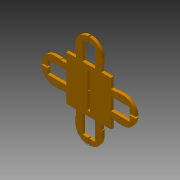
# Autodesk Inventor part: Lock2
Saved by Autodesk Inventor 2014 SP2 (Build 180246200, 246)
## iProperties
Created: 2014-11-24
Part Number: Lock2
Material: Generic
Document SubType Name: Modeling
Designer: JLM
Density: 1 g/cm^3
Appearance: Default
Author: JLM
Autodesk Inventor part; units mm, degrees
ref_plane "YZ Plane" through (0, 0, 0) normal (1, 0, 0) x (0, 1, 0)
ref_plane "XZ Plane" through (0, 0, 0) normal (0, 1, 0) x (-1, 0, 0)
ref_plane "XY Plane" through (0, 0, 0) normal (0, 0, 1) x (1, 0, 0)
sketch "Sketch1" plane through (0, 0, 0) normal (0, 0, 1) x (1, 0, 0)
  line L0 (47.1932, 0) -> (47.1932, 13.335)
  line L1 (47.1932, 13.335) -> (28.1432, 13.335)
  line L2 (28.1432, 13.335) -> (28.1432, 12.7)
  line L3 (28.1432, 12.7) -> (22.4282, 12.7)
  line L4 (12.2521, 0) -> (47.1932, 0)
  line L5 (22.4282, 12.7) -> (22.4282, 22.4282)
  line L6 (22.4282, 22.4282) -> (0, 22.4282)
  line L7 (17.8114, 6.35) -> (17.8114, 0)
  line L8 (47.1932, 0.762) -> (41.275, 0.762)
  line L9 (41.275, 0.762) -> (41.275, 6.35)
  line L10 (41.275, 6.35) -> (17.8114, 6.35)
  line L11 (47.1932, 0) -> (47.1932, -13.335)
  line L12 (47.1932, -13.335) -> (28.1432, -13.335)
  line L13 (28.1432, -13.335) -> (28.1432, -12.7)
  line L14 (28.1432, -12.7) -> (22.4282, -12.7)
  line L15 (22.4282, -12.7) -> (22.4282, -22.4282)
  line L16 (22.4282, -22.4282) -> (0, -22.4282)
  line L17 (17.8114, -6.35) -> (17.8114, 0)
  line L18 (47.1932, -0.762) -> (41.275, -0.762)
  line L19 (41.275, -0.762) -> (41.275, -6.35)
  line L20 (41.275, -6.35) -> (17.8114, -6.35)
  line L21 (0, 22.4282) -> (0, -22.4282)
  point P0 (0, 0)
  dimension "d0" = 13.335
  dimension "d1" = 19.05
  dimension "d6" = 12.7
  dimension "d7" = 22.4282
  dimension "d8" = 22.4282
  dimension "d9" = 5.715
  dimension "d16" = 44.8564
  dimension "d17" = 47.1932
  dimension "d29" = 5.715
  dimension "d31" = 0.762
  constraints: 44 end point, 10 symmetric about line, 7 perpendicular, 4 point on line, 3 parallel
  measures "d0" distance of L0.start L0.end
  measures "d1" distance of L0.end L1.end
  measures "d6" distance between parallel lines of L4 L3
  measures "d7" distance between parallel lines of L4 L6
  measures "d8" distance from line of L5 point (0, 0)
  measures "d9" distance of L2.end L3.end
  measures "d16" distance between parallel lines of L16 L6
  measures "d17" distance from line of L11 point (0, 0)
  measures "d29" distance of L14.start L15.start
  measures "d31" distance between parallel lines of L4 L8
extrude "Extrusion2" add sketch "Sketch1" along normal blind 2.794 contours L8 L9 L10 L7 L17 L20 L19 L18 L11 L12 L13 L14 L15 L16 L21 L6 L5 L3 L2 L1 L0
pattern_circular "Circular Pattern1" count 4 over 360 about axis through (0, 0, -10) along (0, 0, 1) of "Extrusion2"
fillet "Fillet2" radius 12.7 2 edges at (47.1932, 13.335, 1.397) (47.1932, -13.335, 1.397)
fillet "Fillet3" radius 12.7 6 edges at (-47.1932, -13.335, 1.397) (-47.1932, 13.335, 1.397) (-13.335, 47.1932, 1.397) (13.335, 47.1932, 1.397) (-13.335, -47.1932, 1.397) (13.335, -47.1932, 1.397)
sketch "Sketch2" plane through (0, 0, 2.794) normal (0, 0, 1) x (1, 0, 0)
  line L0 (-1.27, -17.526) -> (1.27, -17.526)
  line L1 (1.27, -17.526) -> (1.27, 17.526)
  line L2 (1.27, 17.526) -> (-1.27, 17.526)
  line L3 (-1.27, 17.526) -> (-1.27, -17.526)
  line L4 (-1.27, -17.526) -> (1.27, 17.526) construction
  line L5 (1.27, -17.526) -> (-1.27, 17.526) construction
  point P0 (0, 0)
  dimension "d23" = 2.54
  dimension "d24" = 35.052
  constraints: 12 end point, 2 midpoint, 2 parallel, 1 horizontal, 1 perpendicular
  measures "d23" distance of L2.end L1.end
  measures "d24" distance of L1.end L0.end
extrude "Extrusion3" cut sketch "Sketch2" against normal up to next
equation "\"d7\" = d8"
body "Solid2"
